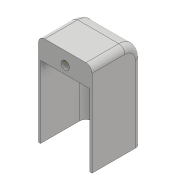
# Autodesk Inventor part: little_rays_shell
Saved by Autodesk Inventor 2017 (Build 210142000, 142)
## iProperties
Created: 2018-04-26
Part Number: little_rays_shell
Material: Generic
Document SubType Name: Modeling
Designer: mfans
Density: 1 g/cm^3
Appearance: Default
Author: mfans
Autodesk Inventor part; units mm, degrees
ref_plane "YZ Plane" through (0, 0, 0) normal (1, 0, 0) x (0, 1, 0)
ref_plane "XZ Plane" through (0, 0, 0) normal (0, 1, 0) x (-1, 0, 0)
ref_plane "XY Plane" through (0, 0, 0) normal (0, 0, 1) x (1, 0, 0)
sketch "Sketch1" plane through (0, 0, 0) normal (0, 1, 0) x (-1, 0, 0)
  line L0 (-13, -5) -> (13, -5)
  line L1 (13, -5) -> (13, 5)
  line L2 (13, 5) -> (-13, 5)
  line L3 (-13, 5) -> (-13, -5)
  line L4 (-13, -5) -> (13, 5) construction
  line L5 (13, -5) -> (-13, 5) construction
  point P0 (0, 0)
  dimension "d0" = 26
  dimension "d1" = 10
  constraints: 12 end point, 2 midpoint, 2 parallel, 1 horizontal, 1 perpendicular
  measures "d0" distance of L1.end L2.end
  measures "d1" distance of L0.end L1.end
extrude "Extrusion1" add sketch "Sketch1" along normal blind 14
sketch "Sketch2" plane through (0, 0, 0) normal (0, -1, 0) x (1, 0, 0)
  line L0 (13, -5) -> (-13, -5) projected
  line L1 (13, 5) -> (13, -5) projected
  line L2 (-13, 5) -> (13, 5) projected
  line L3 (-13, -5) -> (-13, 5) projected
  line L4 (-4.5, 3) -> (4.5, 3)
  line L5 (4.5, 3) -> (4.5, -5)
  line L6 (4.5, -5) -> (-4.5, -5)
  line L7 (-4.5, -5) -> (-4.5, 3)
  line L8 (-4.5, 3) -> (4.5, -5) construction
  line L9 (4.5, 3) -> (-4.5, -5) construction
  point P0 (0, 0)
  point P1 (0, -1)
  dimension "d4" = 9
  dimension "d5" = 4.5
  dimension "d6" = 8
  constraints: 12 end point, 2 midpoint, 2 parallel, 1 horizontal, 1 perpendicular, 1 point on line
  measures "d4" distance of L4.start L4.end
  measures "d5" distance from line of point (0, 0) L5
  measures "d6" distance of L4.end L5.end
extrude "Extrusion2" cut sketch "Sketch2" against normal blind 3 contours L0 L7 L4 L5
fillet "Fillet1" radius 3 2 edges at (-4.5, 1.5, -5) (4.5, 1.5, -5)
sketch "Sketch3" plane through (0, 3, 0) normal (0, -1, 0) x (1, 0, 0)
  line L0 (-4.5, 3) -> (4.5, 3) projected
  point P0 (0, 0)
  point P1 (0, -1.1)
  dimension "d10" = 4.1
  measures "d10" distance from line of L0 point (0, -1.1)
hole "Hole1" at (0, 3, -1.1) direction (0, 1, 0) diameter 4 end through all
sketch "Sketch4" plane through (13, 14, -5) normal (0, 0, -1) x (-1, 0, 0)
  line L0 (5.5, -11) -> (20.5, -11) projected
  line L1 (20.5, -14) -> (20.5, -11) projected
  line L2 (20.5, -14) -> (26, -14) projected
  line L3 (26, -14) -> (26, 0) projected
  line L4 (0, 0) -> (26, 0) projected
  line L5 (0, -14) -> (0, 0) projected
  line L6 (0, -14) -> (5.5, -14) projected
  line L7 (5.5, -11) -> (5.5, -14) projected
  line L8 (0, -14) -> (0, 0) projected
  line L9 (0, -14) -> (1, -14)
  line L10 (1, -14) -> (1, 0)
  line L11 (1, 0) -> (0, 0)
  line L12 (0, 0) -> (0, -14)
  line L13 (20.5, -14) -> (26, -14) projected
  line L14 (26, -14) -> (25, -14)
  line L15 (25, -14) -> (25, 0)
  line L16 (25, 0) -> (26, 0)
  line L17 (26, 0) -> (26, -14)
  line L18 (1, -2) -> (25, -2)
  line L19 (25, -2) -> (25, 0)
  line L20 (25, 0) -> (1, 0)
  line L21 (1, 0) -> (1, -2)
  point P0 (13, -14)
  dimension "d18" = 1
  dimension "d19" = 1
  dimension "d20" = 2
  constraints: 24 end point, 6 parallel, 3 horizontal, 3 perpendicular, 3 point on line
  measures "d18" distance between parallel lines of L5 L10
  measures "d19" distance between parallel lines of L15 L3
  measures "d20" distance between parallel lines of L4 L18
extrude "Extrusion3" add sketch "Sketch4" along normal blind 35 contours L6 L5 L4 L10 | L15 L4 L3 L2 | L10 L4 L15 L18
sketch "Sketch5" plane through (0, 14, 0) normal (0, 1, 0) x (1, 0, 0)
  circle A0 centre (0, 1.1) radius 2 projected
  circle A1 centre (0, 1.1) radius 3
  point P0 (0, 0)
  dimension "d23" = 6
  constraints: 1 centre point, 1 coincident
  measures "d23" diameter of A1
extrude "Extrusion4" cut sketch "Sketch5" against normal blind 2
fillet "Fillet2" radius 8 1 edges at (0, 14, 5)
sketch "Sketch6" plane through (0, 0, 0) normal (0, -1, 0) x (1, 0, 0)
  arc A0 (4.5, -2) -> (7.5, -5) centre (7.5, -2) ccw projected
  line L0 (12, -5) -> (7.5, -5) projected
  line L1 (12, -5) -> (12, -40) projected
  line L2 (13, -40) -> (12, -40) projected
  line L3 (13, 5) -> (13, -40) projected
  line L4 (-13, 5) -> (13, 5) projected
  line L5 (-13, 5) -> (-13, -40) projected
  line L6 (-12, -40) -> (-13, -40) projected
  line L7 (-12, -5) -> (-12, -40) projected
  line L8 (-7.5, -5) -> (-12, -5) projected
  arc A1 (-7.5, -5) -> (-4.5, -2) centre (-7.5, -2) ccw projected
  line L9 (-4.5, -2) -> (-4.5, 3) projected
  line L10 (-4.5, 3) -> (4.5, 3) projected
  line L11 (4.5, 3) -> (4.5, -2) projected
  point P0 (0, 0)
extrude "Extrusion5" add sketch "Sketch6" along normal blind 10
fillet "Fillet3" radius 3 2 edges at (12, 12, -22.5) (-12, 12, -22.5)
fillet "Fillet4" radius 3 6 edges at (13, 11.6569, 2.6569) (13, -2, 5) (13, 14, -21.5) (-13, 11.6569, 2.6569) (-13, -2, 5) (-13, 14, -21.5)
sketch "Sketch7" plane through (0, -10, 0) normal (0, -1, 0) x (1, 0, 0)
  point P0 (0, 0)
sketch "Sketch8" plane through (0, -10, 0) normal (0, -1, 0) x (1, 0, 0)
  line L0 (9.9543, -5) -> (-10.0457, -5)
  line L1 (-10.0457, -5) -> (-10.0457, 4.3303)
  line L2 (-10.0457, 4.3303) -> (9.9543, 4.3303)
  line L3 (9.9543, 4.3303) -> (9.9543, -5)
  line L4 (7.5, -5) -> (-7.5, -5) projected
  point P0 (0, 0)
  dimension "d33" = 20
  dimension "d34" = 0
  constraints: 8 end point, 2 parallel, 1 horizontal, 1 perpendicular
  measures "d33" distance of L1.end L2.end
  measures "d34" distance between parallel lines of L4 L0
extrude "Extrusion6" add sketch "Sketch8" against normal blind 9.5
sketch "Sketch9" plane through (0, 3, 0) normal (0, -1, 0) x (1, 0, 0)
  circle A0 centre (0, -1.1) radius 2 projected
  point P0 (0, 0)
extrude "Extrusion7" cut sketch "Sketch9" along normal through all
body "Solid1"
